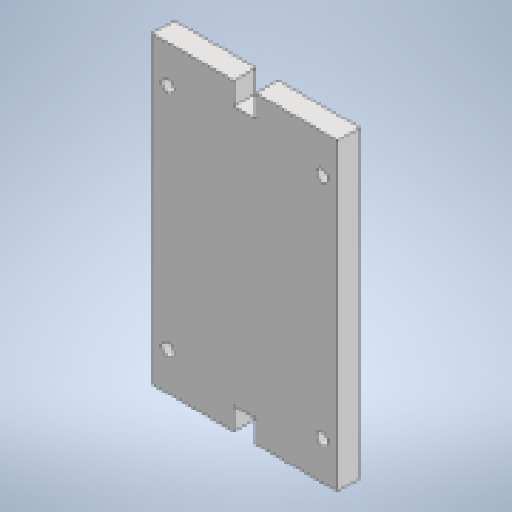
# Autodesk Inventor part: head_up
Saved by Autodesk Inventor 2024 (Build 280153000, 153)
## iProperties
Created: 2024-09-18
Part Number: head_up
Material: 일반
Document SubType Name: Modeling
Designer: Eungang
Density: 1 g/cm^3
Appearance: 기본값
Author: Eungang
Autodesk Inventor part; units mm, degrees
ref_plane "YZ Plane" through (0, 0, 0) normal (1, 0, 0) x (0, 1, 0)
ref_plane "XZ Plane" through (0, 0, 0) normal (0, 1, 0) x (-1, 0, 0)
ref_plane "XY Plane" through (0, 0, 0) normal (0, 0, 1) x (1, 0, 0)
sketch "스케치1" plane through (0, 0, 0) normal (0, 0, 1) x (1, 0, 0)
  line L0 (0, 0) -> (22, 0) projected
  line L1 (0, 6) -> (22, 6) projected
  line L2 (0, -76) -> (22, -76) projected
  line L3 (0, -70) -> (22, -70) projected
  line L4 (0, 6) -> (50, 6)
  line L5 (50, 6) -> (50, -76)
  line L6 (50, -76) -> (0, -76)
  line L7 (0, -76) -> (0, 6)
  line L8 (22, 0) -> (28, 0) projected
  line L9 (28, 0) -> (28, 6) projected
  line L10 (22, 6) -> (22, 0) projected
  line L11 (22, -76) -> (28, -76) projected
  line L12 (28, -76) -> (28, -70) projected
  line L13 (22, -70) -> (22, -76) projected
  line L14 (22, 0) -> (22, 6) projected
  line L15 (28, 6) -> (22, 6) projected
  line L16 (28, -70) -> (22, -70) projected
  line L17 (22, -76) -> (22, -70) projected
  line L18 (0, -76) -> (0, -70) projected
  line L19 (0, 0) -> (0, 6) projected
  line L20 (22, 6.2) -> (28.2, 6.2)
  line L21 (28.2, 6.2) -> (28.2, -0.2)
  line L22 (28.2, -0.2) -> (22, -0.2)
  line L23 (21.8, 6) -> (21.8, 0)
  line L24 (21.8, 0) -> (21.8, -0.2)
  line L25 (21.8, -0.2) -> (22, -0.2)
  line L26 (21.8, 6) -> (21.8, 6.2)
  line L27 (21.8, 6.2) -> (22, 6.2)
  line L28 (50, -35) -> (45, -35)
  line L29 (22, -70) -> (28, -70)
  line L30 (28, -70) -> (28, -76)
  line L31 (22, -76) -> (22, -70)
  line L32 (22, -70) -> (22, -76)
  line L33 (28, -76) -> (22, -76)
  line L34 (22, -76.2) -> (28.2, -76.2)
  line L35 (28.2, -76.2) -> (28.2, -69.8)
  line L36 (28.2, -69.8) -> (22, -69.8)
  line L37 (21.8, -76) -> (21.8, -70)
  line L38 (21.8, -70) -> (21.8, -69.8)
  line L39 (21.8, -69.8) -> (22, -69.8)
  line L40 (21.8, -76) -> (21.8, -76.2)
  line L41 (21.8, -76.2) -> (22, -76.2)
  circle A0 centre (28.2, -0.2) radius 1
  circle A1 centre (21.8, -0.2) radius 1
  circle A2 centre (28.2, 6.2) radius 1
  circle A3 centre (21.8, 6.2) radius 1
  circle A4 centre (28.2, -69.8) radius 1
  circle A5 centre (21.8, -69.8) radius 1
  circle A6 centre (28.2, -76.2) radius 1
  circle A7 centre (21.8, -76.2) radius 1
  point P0 (50, -70)
  point P1 (50, 0)
  point P2 (28.2, -76)
  point P3 (28.2, 6)
  dimension "d7" = 0.2
  dimension "d8" = 0.2
  dimension "d9" = 2
  dimension "d10" = 2
  dimension "d11" = 2
  dimension "d12" = 2
  constraints: 52 end point, 12 symmetric about line, 8 centre point, 4 coincident, 3 parallel, 3 perpendicular, 2 horizontal, 2 point on line, 1 midpoint, 1 vertical, 6 other
  measures "d7" distance between parallel lines of L9 L21
  measures "d8" distance between parallel lines of L10 L23
  measures "d9" diameter of A0
  measures "d10" diameter of A1
  measures "d11" diameter of A2
  measures "d12" diameter of A3
extrude "돌출1" add sketch "스케치1" along normal blind 6 contours L24 L25 L22 A1 L0 | L0 A1 L23 | A1 L22 A0 L21 A2 L4 L5 L6 A6 L35 A4 L36 A5 L3 L7 L0 | L0 L7 L1 A3 L23 A1 | A3 L1 L23 | L3 A5 L37 A7 L2 L7 | L22 L21 A0 | A5 L36 L39 L38 L3 | L3 L37 A5 | A7 L37 L2 | L21 L4 A2 | A4 L35 L36 | L2 L6 A7 L34 L41 L40 | A7 L6 A6 L34 | A6 L6 L35 L34 | A6 L6 L35 picked at (27.8, -76.1333)
sketch "스케치2" plane through (0, 0, 6) normal (0, 0, 1) x (1, 0, 0)
  circle A0 centre (45.8, -4.2) radius 1.6 projected
  circle A1 centre (45.8, -65.8) radius 1.6 projected
  circle A2 centre (4.2, -4.2) radius 1.6 projected
  circle A3 centre (4.2, -65.8) radius 1.6 projected
  line L0 (50, -70) -> (50, 0) projected
  line L1 (50, 0) -> (0, 0) projected
  line L2 (0, 0) -> (0, -70) projected
  line L3 (0, -70) -> (50, -70) projected
  line L4 (28.4609, -19.5584) -> (28.4609, -20.3691) projected
  line L5 (28.4609, -20.3691) -> (23.0826, -20.3691) projected
  line L6 (23.0826, -20.3691) -> (23.0826, -22.4156) projected
  line L7 (23.0826, -22.4156) -> (22.3609, -22.4156) projected
  line L8 (22.3609, -22.4156) -> (22.3609, -17.5118) projected
  line L9 (22.3609, -17.5118) -> (23.0826, -17.5118) projected
  line L10 (23.0826, -17.5118) -> (23.0826, -19.5584) projected
  line L11 (23.0826, -19.5584) -> (28.4609, -19.5584) projected
  spline S0 degree 2 poles (28.0259, -26.6668) (28.3126, -26.9584) (28.5894, -27.7296) (28.5894, -28.2931) knots 0 0 0 1 2 2 2 projected
  spline S1 degree 2 poles (28.5894, -28.2931) (28.5894, -28.8319) (28.3076, -29.6328) (28.0259, -29.9145) knots 0 0 0 1 2 2 2 projected
  spline S2 degree 2 poles (28.0259, -29.9145) (27.7095, -30.2358) (26.8197, -30.4978) (26.1672, -30.4978) knots 0 0 0 1 2 2 2 projected
  line L12 (26.1672, -30.4978) -> (22.3609, -30.4978) projected
  line L13 (22.3609, -30.4978) -> (22.3609, -29.6871) projected
  line L14 (22.3609, -29.6871) -> (26.1672, -29.6871) projected
  spline S3 degree 2 poles (26.1672, -29.6871) (26.5923, -29.6871) (27.1657, -29.5784) (27.3981, -29.4251) knots 0 0 0 1 2 2 2 projected
  spline S4 degree 2 poles (27.3981, -29.4251) (27.6452, -29.262) (27.8973, -28.6985) (27.8973, -28.2931) knots 0 0 0 1 2 2 2 projected
  spline S5 degree 2 poles (27.8973, -28.2931) (27.8973, -27.9125) (27.6452, -27.3193) (27.3981, -27.1562) knots 0 0 0 1 2 2 2 projected
  spline S6 degree 2 poles (27.3981, -27.1562) (27.1657, -27.0029) (26.5972, -26.8942) (26.187, -26.8942) knots 0 0 0 1 2 2 2 projected
  line L15 (26.187, -26.8942) -> (22.3609, -26.8942) projected
  line L16 (22.3609, -26.8942) -> (22.3609, -26.0835) projected
  line L17 (22.3609, -26.0835) -> (26.1672, -26.0835) projected
  spline S7 degree 2 poles (26.1672, -26.0835) (26.8049, -26.0835) (27.7144, -26.3405) (28.0259, -26.6668) knots 0 0 0 1 2 2 2 projected
  line L18 (27.838, -41.6696) -> (28.4609, -41.6696) projected
  line L19 (28.4609, -41.6696) -> (28.4609, -44.0325) projected
  line L20 (28.4609, -44.0325) -> (27.838, -44.0325) projected
  line L21 (27.838, -44.0325) -> (27.838, -43.2564) projected
  line L22 (27.838, -43.2564) -> (22.9837, -43.2564) projected
  line L23 (22.9837, -43.2564) -> (22.9837, -44.0325) projected
  line L24 (22.9837, -44.0325) -> (22.3609, -44.0325) projected
  line L25 (22.3609, -44.0325) -> (22.3609, -41.6696) projected
  line L26 (22.3609, -41.6696) -> (22.9837, -41.6696) projected
  line L27 (22.9837, -41.6696) -> (22.9837, -42.4457) projected
  line L28 (22.9837, -42.4457) -> (27.838, -42.4457) projected
  line L29 (27.838, -42.4457) -> (27.838, -41.6696) projected
  spline S8 degree 2 poles (28.3917, -45.3623) (28.4806, -45.6292) (28.5696, -46.084) (28.5696, -46.4498) knots 0 0 0 1 2 2 2 projected
  spline S9 degree 2 poles (28.5696, -46.4498) (28.5696, -47.043) (28.1692, -48.0464) (27.7688, -48.4123) knots 0 0 0 1 2 2 2 projected
  spline S10 degree 2 poles (27.7688, -48.4123) (27.3733, -48.7781) (26.187, -49.1785) (25.4158, -49.1785) knots 0 0 0 1 2 2 2 projected
  spline S11 degree 2 poles (25.4158, -49.1785) (24.6496, -49.1785) (23.5126, -48.7879) (23.0925, -48.4172) knots 0 0 0 1 2 2 2 projected
  spline S12 degree 2 poles (23.0925, -48.4172) (22.6822, -48.0514) (22.2521, -47.0529) (22.2521, -46.4349) knots 0 0 0 1 2 2 2 projected
  spline S13 degree 2 poles (22.2521, -46.4349) (22.2521, -46.1285) (22.3411, -45.5896) (22.4103, -45.3623) knots 0 0 0 1 2 2 2 projected
  spline S14 degree 2 poles (22.4103, -45.3623) (22.4746, -45.1645) (22.6575, -44.7542) (22.7662, -44.5516) knots 0 0 0 1 2 2 2 projected
  line L30 (22.7662, -44.5516) -> (23.745, -44.5516) projected
  line L31 (23.745, -44.5516) -> (23.745, -44.6158) projected
  spline S15 degree 2 poles (23.745, -44.6158) (23.6461, -44.7246) (23.3693, -45.0607) (23.2358, -45.3029) knots 0 0 0 1 2 2 2 projected
  spline S16 degree 2 poles (23.2358, -45.3029) (23.1073, -45.5353) (22.9442, -46.084) (22.9442, -46.4399) knots 0 0 0 1 2 2 2 projected
  spline S17 degree 2 poles (22.9442, -46.4399) (22.9442, -46.8304) (23.2655, -47.5274) (23.572, -47.7894) knots 0 0 0 1 2 2 2 projected
  spline S18 degree 2 poles (23.572, -47.7894) (23.8834, -48.0464) (24.8276, -48.3332) (25.4158, -48.3332) knots 0 0 0 1 2 2 2 projected
  spline S19 degree 2 poles (25.4158, -48.3332) (26.0436, -48.3332) (26.9482, -48.0316) (27.2596, -47.7696) knots 0 0 0 1 2 2 2 projected
  spline S20 degree 2 poles (27.2596, -47.7696) (27.5612, -47.5126) (27.8677, -46.8255) (27.8677, -46.4399) knots 0 0 0 1 2 2 2 projected
  spline S21 degree 2 poles (27.8677, -46.4399) (27.8677, -46.0889) (27.6947, -45.4908) (27.5661, -45.2584) knots 0 0 0 1 2 2 2 projected
  spline S22 degree 2 poles (27.5661, -45.2584) (27.4376, -45.036) (27.1707, -44.7048) (27.0767, -44.6109) knots 0 0 0 1 2 2 2 projected
  line L32 (27.0767, -44.6109) -> (27.0767, -44.5516) projected
  line L33 (27.0767, -44.5516) -> (28.0456, -44.5516) projected
  spline S23 degree 2 poles (28.0456, -44.5516) (28.1396, -44.7542) (28.3126, -45.1101) (28.3917, -45.3623) knots 0 0 0 1 2 2 2 projected
  line L34 (25.8063, -38.1154) -> (28.4609, -35.9453) projected
  line L35 (28.4609, -35.9453) -> (28.4609, -36.9982) projected
  line L36 (28.4609, -36.9982) -> (26.0337, -38.9261) projected
  line L37 (26.0337, -38.9261) -> (26.0337, -39.8554) projected
  line L38 (26.0337, -39.8554) -> (28.4609, -39.8554) projected
  line L39 (28.4609, -39.8554) -> (28.4609, -40.6661) projected
  line L40 (28.4609, -40.6661) -> (22.3609, -40.6661) projected
  line L41 (22.3609, -40.6661) -> (22.3609, -39.0942) projected
  spline S24 degree 2 poles (22.3609, -39.0942) (22.3609, -38.5702) (22.4746, -37.8633) (22.6822, -37.542) knots 0 0 0 1 2 2 2 projected
  spline S25 degree 2 poles (22.6822, -37.542) (22.8898, -37.2207) (23.5374, -36.8499) (24.0169, -36.8499) knots 0 0 0 1 2 2 2 projected
  spline S26 degree 2 poles (24.0169, -36.8499) (24.6842, -36.8499) (25.5888, -37.5321) (25.8063, -38.1154) knots 0 0 0 1 2 2 2 projected
  spline S27 degree 2 poles (28.3917, -31.9907) (28.4806, -32.2576) (28.5696, -32.7124) (28.5696, -33.0782) knots 0 0 0 1 2 2 2 projected
  spline S28 degree 2 poles (28.5696, -33.0782) (28.5696, -33.6714) (28.1692, -34.6749) (27.7688, -35.0407) knots 0 0 0 1 2 2 2 projected
  spline S29 degree 2 poles (27.7688, -35.0407) (27.3733, -35.4065) (26.187, -35.8069) (25.4158, -35.8069) knots 0 0 0 1 2 2 2 projected
  spline S30 degree 2 poles (25.4158, -35.8069) (24.6496, -35.8069) (23.5126, -35.4164) (23.0925, -35.0456) knots 0 0 0 1 2 2 2 projected
  spline S31 degree 2 poles (23.0925, -35.0456) (22.6822, -34.6798) (22.2521, -33.6813) (22.2521, -33.0634) knots 0 0 0 1 2 2 2 projected
  spline S32 degree 2 poles (22.2521, -33.0634) (22.2521, -32.7569) (22.3411, -32.2181) (22.4103, -31.9907) knots 0 0 0 1 2 2 2 projected
  spline S33 degree 2 poles (22.4103, -31.9907) (22.4746, -31.793) (22.6575, -31.3827) (22.7662, -31.18) knots 0 0 0 1 2 2 2 projected
  line L42 (22.7662, -31.18) -> (23.745, -31.18) projected
  line L43 (23.745, -31.18) -> (23.745, -31.2443) projected
  spline S34 degree 2 poles (23.745, -31.2443) (23.6461, -31.353) (23.3693, -31.6892) (23.2358, -31.9314) knots 0 0 0 1 2 2 2 projected
  spline S35 degree 2 poles (23.2358, -31.9314) (23.1073, -32.1637) (22.9442, -32.7124) (22.9442, -33.0683) knots 0 0 0 1 2 2 2 projected
  spline S36 degree 2 poles (22.9442, -33.0683) (22.9442, -33.4588) (23.2655, -34.1558) (23.572, -34.4178) knots 0 0 0 1 2 2 2 projected
  spline S37 degree 2 poles (23.572, -34.4178) (23.8834, -34.6749) (24.8276, -34.9616) (25.4158, -34.9616) knots 0 0 0 1 2 2 2 projected
  spline S38 degree 2 poles (25.4158, -34.9616) (26.0436, -34.9616) (26.9482, -34.6601) (27.2596, -34.3981) knots 0 0 0 1 2 2 2 projected
  spline S39 degree 2 poles (27.2596, -34.3981) (27.5612, -34.141) (27.8677, -33.4539) (27.8677, -33.0683) knots 0 0 0 1 2 2 2 projected
  spline S40 degree 2 poles (27.8677, -33.0683) (27.8677, -32.7174) (27.6947, -32.1192) (27.5661, -31.8869) knots 0 0 0 1 2 2 2 projected
  spline S41 degree 2 poles (27.5661, -31.8869) (27.4376, -31.6644) (27.1707, -31.3332) (27.0767, -31.2393) knots 0 0 0 1 2 2 2 projected
  line L44 (27.0767, -31.2393) -> (27.0767, -31.18) projected
  line L45 (27.0767, -31.18) -> (28.0456, -31.18) projected
  spline S42 degree 2 poles (28.0456, -31.18) (28.1396, -31.3827) (28.3126, -31.7386) (28.3917, -31.9907) knots 0 0 0 1 2 2 2 projected
  line L46 (27.838, -22.7962) -> (28.4609, -22.7962) projected
  line L47 (28.4609, -22.7962) -> (28.4609, -25.1591) projected
  line L48 (28.4609, -25.1591) -> (27.838, -25.1591) projected
  line L49 (27.838, -25.1591) -> (27.838, -24.383) projected
  line L50 (27.838, -24.383) -> (22.9837, -24.383) projected
  line L51 (22.9837, -24.383) -> (22.9837, -25.1591) projected
  line L52 (22.9837, -25.1591) -> (22.3609, -25.1591) projected
  line L53 (22.3609, -25.1591) -> (22.3609, -22.7962) projected
  line L54 (22.3609, -22.7962) -> (22.9837, -22.7962) projected
  line L55 (22.9837, -22.7962) -> (22.9837, -23.5723) projected
  line L56 (22.9837, -23.5723) -> (27.838, -23.5723) projected
  line L57 (27.838, -23.5723) -> (27.838, -22.7962) projected
extrude "돌출2" cut sketch "스케치2" against normal blind 6 contours A0 | A1 | A2 | A3
sketch "스케치3" plane through (0, 0, 6) normal (0, 0, 1) x (1, 0, 0)
  circle A0 centre (4.2, -65.8) radius 1.6 projected
  circle A1 centre (45.8, -65.8) radius 1.6 projected
  circle A2 centre (4.2, -4.2) radius 1.6 projected
  circle A3 centre (45.8, -4.2) radius 1.6 projected
  line L0 (50, 6) -> (28.2, 6) projected
  line L1 (21.8, 6) -> (0, 6) projected
  line L2 (0, 6) -> (0, -76) projected
  line L3 (0, -76) -> (21.8, -76) projected
  line L4 (50, -76) -> (50, 6) projected
  line L5 (28, 3) -> (45.8, 3)
  circle A4 centre (45.8, 3) radius 1.35
  line L6 (25, 0) -> (25, 3)
  circle A5 centre (4.2, 3) radius 1.35
  line L7 (50, -35) -> (44.45, -35)
  circle A6 centre (45.8, -73) radius 1.35
  circle A7 centre (4.2, -73) radius 1.35
  line L8 (28.2, -76.2) -> (28.2, -76) projected
  line L9 (28.2, -76) -> (21.8, -76) projected
  line L10 (21.8, -76) -> (21.8, -76.2) projected
  line L11 (21.8, -76.2) -> (28.2, -76.2) projected
  line L12 (28.2, -0.2) -> (21.8, -0.2) projected
  line L13 (21.8, -0.2) -> (21.8, 6) projected
  line L14 (21.8, -76) -> (21.8, -69.8) projected
  line L15 (21.8, -69.8) -> (28.2, -69.8) projected
  line L16 (28.2, -69.8) -> (28.2, -76) projected
  line L17 (28.2, -76) -> (50, -76) projected
  line L18 (28.2, 6) -> (28.2, -0.2) projected
  point P0 (0, 0)
  dimension "d4" = 2.7
  constraints: 6 end point, 4 centre point, 3 symmetric about line, 2 horizontal, 1 coincident, 1 midpoint, 1 vertical, 3 other
  measures "d4" diameter of A4
extrude "돌출3" cut sketch "스케치3" against normal up to next contours A4 | L8 L11 L10 L9 | A5 | A6 | A7
